Autodesk Fusion 360 part; units mm, degrees
(part 2 of 8)
  line L951 (106.594, 69.8334) -> (107.395, 69.8334)
  line L952 (107.395, 69.8334) -> (107.395, 64.0334)
  line L953 (107.395, 64.0334) -> (106.594, 64.0334)
  line L954 (106.594, 64.0334) -> (106.594, 60.9328)
  line L955 (106.594, 60.9328) -> (107.395, 60.9328)
  line L956 (107.395, 60.9328) -> (107.395, 59.9338)
  line L957 (107.395, 59.9338) -> (121.394, 59.9338)
  line L958 (121.394, 59.9338) -> (121.394, 60.9328)
  line L959 (121.394, 60.9328) -> (122.195, 60.9328)
  line L960 (122.195, 60.9328) -> (122.195, 64.0334)
  line L961 (122.195, 64.0334) -> (121.394, 64.0334)
  line L962 (121.394, 64.0334) -> (121.394, 69.8334)
  line L963 (121.394, 69.8334) -> (122.195, 69.8334)
  line L964 (122.195, 69.8334) -> (122.195, 72.9326)
  line L965 (122.195, 72.9326) -> (121.394, 72.9326)
  line L966 (121.394, 72.9326) -> (121.394, 73.9331)
  line L967 (121.394, 73.9331) -> (107.395, 73.9331)
  line L968 (126.445, 73.9331) -> (126.445, 72.9326)
  line L969 (126.445, 72.9326) -> (125.644, 72.9326)
  line L970 (125.644, 72.9326) -> (125.644, 69.8334)
  line L971 (125.644, 69.8334) -> (126.445, 69.8334)
  line L972 (126.445, 69.8334) -> (126.445, 64.0334)
  line L973 (126.445, 64.0334) -> (125.644, 64.0334)
  line L974 (125.644, 64.0334) -> (125.644, 60.9328)
  line L975 (125.644, 60.9328) -> (126.445, 60.9328)
  line L976 (126.445, 60.9328) -> (126.445, 59.9338)
  line L977 (126.445, 59.9338) -> (140.444, 59.9338)
  line L978 (140.444, 59.9338) -> (140.444, 60.9328)
  line L979 (140.444, 60.9328) -> (141.245, 60.9328)
  line L980 (141.245, 60.9328) -> (141.245, 64.0334)
  line L981 (141.245, 64.0334) -> (140.444, 64.0334)
  line L982 (140.444, 64.0334) -> (140.444, 69.8334)
  line L983 (140.444, 69.8334) -> (141.245, 69.8334)
  line L984 (141.245, 69.8334) -> (141.245, 72.9326)
  line L985 (141.245, 72.9326) -> (140.444, 72.9326)
  line L986 (140.444, 72.9326) -> (140.444, 73.9331)
  line L987 (140.444, 73.9331) -> (126.445, 73.9331)
  line L988 (145.495, 73.9331) -> (145.495, 72.9326)
  line L989 (145.495, 72.9326) -> (144.694, 72.9326)
  line L990 (144.694, 72.9326) -> (144.694, 69.8334)
  line L991 (144.694, 69.8334) -> (145.495, 69.8334)
  line L992 (145.495, 69.8334) -> (145.495, 64.0334)
  line L993 (145.495, 64.0334) -> (144.694, 64.0334)
  line L994 (144.694, 64.0334) -> (144.694, 60.9328)
  line L995 (144.694, 60.9328) -> (145.495, 60.9328)
  line L996 (145.495, 60.9328) -> (145.495, 59.9338)
  line L997 (145.495, 59.9338) -> (159.494, 59.9338)
  line L998 (159.494, 59.9338) -> (159.494, 60.9328)
  line L999 (159.494, 60.9328) -> (160.295, 60.9328)
  line L1000 (160.295, 60.9328) -> (160.295, 64.0334)
  line L1001 (160.295, 64.0334) -> (159.494, 64.0334)
  line L1002 (159.494, 64.0334) -> (159.494, 69.8334)
  line L1003 (159.494, 69.8334) -> (160.295, 69.8334)
  line L1004 (160.295, 69.8334) -> (160.295, 72.9326)
  line L1005 (160.295, 72.9326) -> (159.494, 72.9326)
  line L1006 (159.494, 72.9326) -> (159.494, 73.9331)
  line L1007 (159.494, 73.9331) -> (145.495, 73.9331)
  line L1008 (164.545, 73.9331) -> (164.545, 72.9326)
  line L1009 (164.545, 72.9326) -> (163.744, 72.9326)
  line L1010 (163.744, 72.9326) -> (163.744, 69.8334)
  line L1011 (163.744, 69.8334) -> (164.545, 69.8334)
  line L1012 (164.545, 69.8334) -> (164.545, 64.0334)
  line L1013 (164.545, 64.0334) -> (163.744, 64.0334)
  line L1014 (163.744, 64.0334) -> (163.744, 60.9328)
  line L1015 (163.744, 60.9328) -> (164.545, 60.9328)
  line L1016 (164.545, 60.9328) -> (164.545, 59.9338)
  line L1017 (164.545, 59.9338) -> (178.544, 59.9338)
  line L1018 (178.544, 59.9338) -> (178.544, 60.9328)
  line L1019 (178.544, 60.9328) -> (179.345, 60.9328)
  line L1020 (179.345, 60.9328) -> (179.345, 64.0334)
  line L1021 (179.345, 64.0334) -> (178.544, 64.0334)
  line L1022 (178.544, 64.0334) -> (178.544, 69.8334)
  line L1023 (178.544, 69.8334) -> (179.345, 69.8334)
  line L1024 (179.345, 69.8334) -> (179.345, 72.9326)
  line L1025 (179.345, 72.9326) -> (178.544, 72.9326)
  line L1026 (178.544, 72.9326) -> (178.544, 73.9331)
  line L1027 (178.544, 73.9331) -> (164.545, 73.9331)
  line L1028 (183.595, 73.9331) -> (183.595, 72.9326)
  line L1029 (183.595, 72.9326) -> (182.794, 72.9326)
  line L1030 (182.794, 72.9326) -> (182.794, 69.8334)
  line L1031 (182.794, 69.8334) -> (183.595, 69.8334)
  line L1032 (183.595, 69.8334) -> (183.595, 64.0334)
  line L1033 (183.595, 64.0334) -> (182.794, 64.0334)
  line L1034 (182.794, 64.0334) -> (182.794, 60.9328)
  line L1035 (182.794, 60.9328) -> (183.595, 60.9328)
  line L1036 (183.595, 60.9328) -> (183.595, 59.9338)
  line L1037 (183.595, 59.9338) -> (197.594, 59.9338)
  line L1038 (197.594, 59.9338) -> (197.594, 60.9328)
  line L1039 (197.594, 60.9328) -> (198.395, 60.9328)
  line L1040 (198.395, 60.9328) -> (198.395, 64.0334)
  line L1041 (198.395, 64.0334) -> (197.594, 64.0334)
  line L1042 (197.594, 64.0334) -> (197.594, 69.8334)
  line L1043 (197.594, 69.8334) -> (198.395, 69.8334)
  line L1044 (198.395, 69.8334) -> (198.395, 72.9326)
  line L1045 (198.395, 72.9326) -> (197.594, 72.9326)
  line L1046 (197.594, 72.9326) -> (197.594, 73.9331)
  line L1047 (197.594, 73.9331) -> (183.595, 73.9331)
  line L1048 (202.645, 73.9331) -> (202.645, 72.9326)
  line L1049 (202.645, 72.9326) -> (201.844, 72.9326)
  line L1050 (201.844, 72.9326) -> (201.844, 69.8334)
  line L1051 (201.844, 69.8334) -> (202.645, 69.8334)
  line L1052 (202.645, 69.8334) -> (202.645, 64.0334)
  line L1053 (202.645, 64.0334) -> (201.844, 64.0334)
  line L1054 (201.844, 64.0334) -> (201.844, 60.9328)
  line L1055 (201.844, 60.9328) -> (202.645, 60.9328)
  line L1056 (202.645, 60.9328) -> (202.645, 59.9338)
  line L1057 (202.645, 59.9338) -> (216.644, 59.9338)
  line L1058 (216.644, 59.9338) -> (216.644, 60.9328)
  line L1059 (216.644, 60.9328) -> (217.445, 60.9328)
  line L1060 (217.445, 60.9328) -> (217.445, 64.0334)
  line L1061 (217.445, 64.0334) -> (216.644, 64.0334)
  line L1062 (216.644, 64.0334) -> (216.644, 69.8334)
  line L1063 (216.644, 69.8334) -> (217.445, 69.8334)
  line L1064 (217.445, 69.8334) -> (217.445, 72.9326)
  line L1065 (217.445, 72.9326) -> (216.644, 72.9326)
  line L1066 (216.644, 72.9326) -> (216.644, 73.9331)
  line L1067 (216.644, 73.9331) -> (202.645, 73.9331)
  line L1068 (221.695, 73.9331) -> (221.695, 72.9326)
  line L1069 (221.695, 72.9326) -> (220.894, 72.9326)
  line L1070 (220.894, 72.9326) -> (220.894, 69.8334)
  line L1071 (220.894, 69.8334) -> (221.695, 69.8334)
  line L1072 (221.695, 69.8334) -> (221.695, 64.0334)
  line L1073 (221.695, 64.0334) -> (220.894, 64.0334)
  line L1074 (220.894, 64.0334) -> (220.894, 60.9328)
  line L1075 (220.894, 60.9328) -> (221.695, 60.9328)
  line L1076 (221.695, 60.9328) -> (221.695, 59.9338)
  line L1077 (221.695, 59.9338) -> (235.694, 59.9338)
  line L1078 (235.694, 59.9338) -> (235.694, 60.9328)
  line L1079 (235.694, 60.9328) -> (236.495, 60.9328)
  line L1080 (236.495, 60.9328) -> (236.495, 64.0334)
  line L1081 (236.495, 64.0334) -> (235.694, 64.0334)
  line L1082 (235.694, 64.0334) -> (235.694, 69.8334)
  line L1083 (235.694, 69.8334) -> (236.495, 69.8334)
  line L1084 (236.495, 69.8334) -> (236.495, 72.9326)
  line L1085 (236.495, 72.9326) -> (235.694, 72.9326)
  line L1086 (235.694, 72.9326) -> (235.694, 73.9331)
  line L1087 (235.694, 73.9331) -> (221.695, 73.9331)
  line L1088 (240.745, 73.9331) -> (240.745, 72.9326)
  line L1089 (240.745, 72.9326) -> (239.944, 72.9326)
  line L1090 (239.944, 72.9326) -> (239.944, 69.8334)
  line L1091 (239.944, 69.8334) -> (240.745, 69.8334)
  line L1092 (240.745, 69.8334) -> (240.745, 64.0334)
  line L1093 (240.745, 64.0334) -> (239.944, 64.0334)
  line L1094 (239.944, 64.0334) -> (239.944, 60.9328)
  line L1095 (239.944, 60.9328) -> (240.745, 60.9328)
  line L1096 (240.745, 60.9328) -> (240.745, 59.9338)
  line L1097 (240.745, 59.9338) -> (254.744, 59.9338)
  line L1098 (254.744, 59.9338) -> (254.744, 60.9328)
  line L1099 (254.744, 60.9328) -> (255.545, 60.9328)
  line L1100 (255.545, 60.9328) -> (255.545, 64.0334)
  line L1101 (255.545, 64.0334) -> (254.744, 64.0334)
  line L1102 (254.744, 64.0334) -> (254.744, 69.8334)
  line L1103 (254.744, 69.8334) -> (255.545, 69.8334)
  line L1104 (255.545, 69.8334) -> (255.545, 72.9326)
  line L1105 (255.545, 72.9326) -> (254.744, 72.9326)
  line L1106 (254.744, 72.9326) -> (254.744, 73.9331)
  line L1107 (254.744, 73.9331) -> (240.745, 73.9331)
  line L1108 (264.557, 73.9331) -> (264.557, 72.9326)
  line L1109 (264.557, 72.9326) -> (263.756, 72.9326)
  line L1110 (263.756, 72.9326) -> (263.756, 69.8334)
  line L1111 (263.756, 69.8334) -> (264.557, 69.8334)
  line L1112 (264.557, 69.8334) -> (264.557, 64.0334)
  line L1113 (264.557, 64.0334) -> (263.756, 64.0334)
  line L1114 (263.756, 64.0334) -> (263.756, 60.9328)
  line L1115 (263.756, 60.9328) -> (264.557, 60.9328)
  line L1116 (264.557, 60.9328) -> (264.557, 59.9338)
  line L1117 (264.557, 59.9338) -> (278.557, 59.9338)
  line L1118 (278.557, 59.9338) -> (278.557, 60.9328)
  line L1119 (278.557, 60.9328) -> (279.356, 60.9328)
  line L1120 (279.356, 60.9328) -> (279.356, 64.0334)
  line L1121 (279.356, 64.0334) -> (278.557, 64.0334)
  line L1122 (278.557, 64.0334) -> (278.557, 69.8334)
  line L1123 (278.557, 69.8334) -> (279.356, 69.8334)
  line L1124 (279.356, 69.8334) -> (279.356, 72.9326)
  line L1125 (279.356, 72.9326) -> (278.557, 72.9326)
  line L1126 (278.557, 72.9326) -> (278.557, 73.9331)
  line L1127 (278.557, 73.9331) -> (264.557, 73.9331)
  line L1128 (293.132, 73.9331) -> (293.132, 72.9326)
  line L1129 (293.132, 72.9326) -> (292.331, 72.9326)
  line L1130 (292.331, 72.9326) -> (292.331, 69.8334)
  line L1131 (292.331, 69.8334) -> (293.132, 69.8334)
  line L1132 (293.132, 69.8334) -> (293.132, 64.0334)
  line L1133 (293.132, 64.0334) -> (292.331, 64.0334)
  line L1134 (292.331, 64.0334) -> (292.331, 60.9328)
  line L1135 (292.331, 60.9328) -> (293.132, 60.9328)
  line L1136 (293.132, 60.9328) -> (293.132, 59.9338)
  line L1137 (293.132, 59.9338) -> (307.132, 59.9338)
  line L1138 (307.132, 59.9338) -> (307.132, 60.9328)
  line L1139 (307.132, 60.9328) -> (307.931, 60.9328)
  line L1140 (307.931, 60.9328) -> (307.931, 64.0334)
  line L1141 (307.931, 64.0334) -> (307.132, 64.0334)
  line L1142 (307.132, 64.0334) -> (307.132, 69.8334)
  line L1143 (307.132, 69.8334) -> (307.931, 69.8334)
  line L1144 (307.931, 69.8334) -> (307.931, 72.9326)
  line L1145 (307.931, 72.9326) -> (307.132, 72.9326)
  line L1146 (307.132, 72.9326) -> (307.132, 73.9331)
  line L1147 (307.132, 73.9331) -> (293.132, 73.9331)
  line L1148 (312.182, 73.9331) -> (312.182, 72.9326)
  line L1149 (312.182, 72.9326) -> (311.381, 72.9326)
  line L1150 (311.381, 72.9326) -> (311.381, 69.8334)
  line L1151 (311.381, 69.8334) -> (312.182, 69.8334)
  line L1152 (312.182, 69.8334) -> (312.182, 64.0334)
  line L1153 (312.182, 64.0334) -> (311.381, 64.0334)
  line L1154 (311.381, 64.0334) -> (311.381, 60.9328)
  line L1155 (311.381, 60.9328) -> (312.182, 60.9328)
  line L1156 (312.182, 60.9328) -> (312.182, 59.9338)
  line L1157 (312.182, 59.9338) -> (326.182, 59.9338)
  line L1158 (326.182, 59.9338) -> (326.182, 60.9328)
  line L1159 (326.182, 60.9328) -> (326.981, 60.9328)
  line L1160 (326.981, 60.9328) -> (326.981, 64.0334)
  line L1161 (326.981, 64.0334) -> (326.182, 64.0334)
  line L1162 (326.182, 64.0334) -> (326.182, 69.8334)
  line L1163 (326.182, 69.8334) -> (326.981, 69.8334)
  line L1164 (326.981, 69.8334) -> (326.981, 72.9326)
  line L1165 (326.981, 72.9326) -> (326.182, 72.9326)
  line L1166 (326.182, 72.9326) -> (326.182, 73.9331)
  line L1167 (326.182, 73.9331) -> (312.182, 73.9331)
  line L1168 (259.795, 92.9831) -> (259.795, 91.9826)
  line L1169 (259.795, 91.9826) -> (258.994, 91.9826)
  line L1170 (258.994, 91.9826) -> (258.994, 88.8834)
  line L1171 (258.994, 88.8834) -> (259.795, 88.8834)
  line L1172 (259.795, 88.8834) -> (259.795, 88.2826)
  line L1173 (259.795, 88.2826) -> (258.269, 88.2826)
  line L1174 (258.269, 88.2826) -> (258.269, 91.5127)
  line L1175 (258.269, 91.5127) -> (251.52, 91.5127)
  line L1176 (251.52, 91.5127) -> (251.52, 88.2826)
  line L1177 (251.52, 88.2826) -> (250.694, 88.2826)
  line L1178 (250.694, 88.2826) -> (250.694, 85.4837)
  line L1179 (250.694, 85.4837) -> (251.52, 85.4837)
  line L1180 (251.52, 85.4837) -> (251.52, 79.2138)
  line L1181 (251.52, 79.2138) -> (253.243, 79.2138)
  line L1182 (253.243, 79.2138) -> (253.243, 78.0136)
  line L1183 (253.243, 78.0136) -> (256.544, 78.0136)
  line L1184 (256.544, 78.0136) -> (256.544, 79.2138)
  line L1185 (256.544, 79.2138) -> (258.269, 79.2138)
  line L1186 (258.269, 79.2138) -> (258.269, 83.6828)
  line L1187 (258.269, 83.6828) -> (259.795, 83.6828)
  line L1188 (259.795, 83.6828) -> (259.795, 83.0834)
  line L1189 (259.795, 83.0834) -> (258.994, 83.0834)
  line L1190 (258.994, 83.0834) -> (258.994, 79.9828)
  line L1191 (258.994, 79.9828) -> (259.795, 79.9828)
  line L1192 (259.795, 79.9828) -> (259.795, 78.9838)
  line L1193 (259.795, 78.9838) -> (273.794, 78.9838)
  line L1194 (273.794, 78.9838) -> (273.794, 79.9828)
  line L1195 (273.794, 79.9828) -> (274.595, 79.9828)
  line L1196 (274.595, 79.9828) -> (274.595, 83.0834)
  line L1197 (274.595, 83.0834) -> (273.794, 83.0834)
  line L1198 (273.794, 83.0834) -> (273.794, 83.6828)
  line L1199 (273.794, 83.6828) -> (275.32, 83.6828)
  line L1200 (275.32, 83.6828) -> (275.32, 79.2138)
  line L1201 (275.32, 79.2138) -> (277.045, 79.2138)
  line L1202 (277.045, 79.2138) -> (277.045, 78.0136)
  line L1203 (277.045, 78.0136) -> (280.344, 78.0136)
  line L1204 (280.344, 78.0136) -> (280.344, 79.2138)
  line L1205 (280.344, 79.2138) -> (282.069, 79.2138)
  line L1206 (282.069, 79.2138) -> (282.069, 85.4837)
  line L1207 (282.069, 85.4837) -> (282.895, 85.4837)
  line L1208 (282.895, 85.4837) -> (282.895, 88.2826)
  line L1209 (282.895, 88.2826) -> (282.069, 88.2826)
  line L1210 (282.069, 88.2826) -> (282.069, 91.5127)
  line L1211 (282.069, 91.5127) -> (275.32, 91.5127)
  line L1212 (275.32, 91.5127) -> (275.32, 88.2826)
  line L1213 (275.32, 88.2826) -> (273.794, 88.2826)
  line L1214 (273.794, 88.2826) -> (273.794, 88.8834)
  line L1215 (273.794, 88.8834) -> (274.595, 88.8834)
  line L1216 (274.595, 88.8834) -> (274.595, 91.9826)
  line L1217 (274.595, 91.9826) -> (273.794, 91.9826)
  line L1218 (273.794, 91.9826) -> (273.794, 92.9831)
  line L1219 (273.794, 92.9831) -> (259.795, 92.9831)
  line L1220 (2.6197, 92.9831) -> (2.6197, 91.9826)
  line L1221 (2.6197, 91.9826) -> (1.819, 91.9826)
  line L1222 (1.819, 91.9826) -> (1.819, 88.8834)
  line L1223 (1.819, 88.8834) -> (2.6197, 88.8834)
  line L1224 (2.6197, 88.8834) -> (2.6197, 83.0834)
  line L1225 (2.6197, 83.0834) -> (1.819, 83.0834)
  line L1226 (1.819, 83.0834) -> (1.819, 79.9828)
  line L1227 (1.819, 79.9828) -> (2.6197, 79.9828)
  line L1228 (2.6197, 79.9828) -> (2.6197, 78.9838)
  line L1229 (2.6197, 78.9838) -> (16.6192, 78.9838)
  line L1230 (16.6192, 78.9838) -> (16.6192, 79.9828)
  line L1231 (16.6192, 79.9828) -> (17.4198, 79.9828)
  line L1232 (17.4198, 79.9828) -> (17.4198, 83.0834)
  line L1233 (17.4198, 83.0834) -> (16.6192, 83.0834)
  line L1234 (16.6192, 83.0834) -> (16.6192, 88.8834)
  line L1235 (16.6192, 88.8834) -> (17.4198, 88.8834)
  line L1236 (17.4198, 88.8834) -> (17.4198, 91.9826)
  line L1237 (17.4198, 91.9826) -> (16.6192, 91.9826)
  line L1238 (16.6192, 91.9826) -> (16.6192, 92.9831)
  line L1239 (16.6192, 92.9831) -> (2.6196, 92.9831)
  line L1240 (21.6697, 92.9831) -> (21.6697, 91.9826)
  line L1241 (21.6697, 91.9826) -> (20.869, 91.9826)
  line L1242 (20.869, 91.9826) -> (20.869, 88.8834)
  line L1243 (20.869, 88.8834) -> (21.6697, 88.8834)
  line L1244 (21.6697, 88.8834) -> (21.6697, 83.0834)
  line L1245 (21.6697, 83.0834) -> (20.869, 83.0834)
  line L1246 (20.869, 83.0834) -> (20.869, 79.9828)
  line L1247 (20.869, 79.9828) -> (21.6697, 79.9828)
  line L1248 (21.6697, 79.9828) -> (21.6697, 78.9838)
  line L1249 (21.6697, 78.9838) -> (35.669, 78.9838)
  line L1250 (35.669, 78.9838) -> (35.669, 79.9828)
  line L1251 (35.669, 79.9828) -> (36.4698, 79.9828)
  line L1252 (36.4698, 79.9828) -> (36.4698, 83.0834)
  line L1253 (36.4698, 83.0834) -> (35.669, 83.0834)
  line L1254 (35.669, 83.0834) -> (35.669, 88.8834)
  line L1255 (35.669, 88.8834) -> (36.4698, 88.8834)
  line L1256 (36.4698, 88.8834) -> (36.4698, 91.9826)
  line L1257 (36.4698, 91.9826) -> (35.669, 91.9826)
  line L1258 (35.669, 91.9826) -> (35.669, 92.9831)
  line L1259 (35.669, 92.9831) -> (21.6697, 92.9831)
  line L1260 (40.7197, 92.9831) -> (40.7197, 91.9826)
  line L1261 (40.7197, 91.9826) -> (39.9189, 91.9826)
  line L1262 (39.9189, 91.9826) -> (39.9189, 88.8834)
  line L1263 (39.9189, 88.8834) -> (40.7197, 88.8834)
  line L1264 (40.7197, 88.8834) -> (40.7197, 83.0834)
  line L1265 (40.7197, 83.0834) -> (39.9189, 83.0834)
  line L1266 (39.9189, 83.0834) -> (39.9189, 79.9828)
  line L1267 (39.9189, 79.9828) -> (40.7197, 79.9828)
  line L1268 (40.7197, 79.9828) -> (40.7197, 78.9838)
  line L1269 (40.7197, 78.9838) -> (54.719, 78.9838)
  line L1270 (54.719, 78.9838) -> (54.719, 79.9828)
  line L1271 (54.719, 79.9828) -> (55.5198, 79.9828)
  line L1272 (55.5198, 79.9828) -> (55.5198, 83.0834)
  line L1273 (55.5198, 83.0834) -> (54.719, 83.0834)
  line L1274 (54.719, 83.0834) -> (54.719, 88.8834)
  line L1275 (54.719, 88.8834) -> (55.5198, 88.8834)
  line L1276 (55.5198, 88.8834) -> (55.5198, 91.9826)
  line L1277 (55.5198, 91.9826) -> (54.719, 91.9826)
  line L1278 (54.719, 91.9826) -> (54.719, 92.9831)
  line L1279 (54.719, 92.9831) -> (40.7197, 92.9831)
  line L1280 (59.7697, 92.9831) -> (59.7697, 91.9826)
  line L1281 (59.7697, 91.9826) -> (58.9689, 91.9826)
  line L1282 (58.9689, 91.9826) -> (58.9689, 88.8834)
  line L1283 (58.9689, 88.8834) -> (59.7697, 88.8834)
  line L1284 (59.7697, 88.8834) -> (59.7697, 83.0834)
  line L1285 (59.7697, 83.0834) -> (58.9689, 83.0834)
  line L1286 (58.9689, 83.0834) -> (58.9689, 79.9828)
  line L1287 (58.9689, 79.9828) -> (59.7697, 79.9828)
  line L1288 (59.7697, 79.9828) -> (59.7697, 78.9838)
  line L1289 (59.7697, 78.9838) -> (73.769, 78.9838)
  line L1290 (73.769, 78.9838) -> (73.769, 79.9828)
  line L1291 (73.769, 79.9828) -> (74.5698, 79.9828)
  line L1292 (74.5698, 79.9828) -> (74.5698, 83.0834)
  line L1293 (74.5698, 83.0834) -> (73.769, 83.0834)
  line L1294 (73.769, 83.0834) -> (73.769, 88.8834)
  line L1295 (73.769, 88.8834) -> (74.5698, 88.8834)
  line L1296 (74.5698, 88.8834) -> (74.5698, 91.9826)
  line L1297 (74.5698, 91.9826) -> (73.769, 91.9826)
  line L1298 (73.769, 91.9826) -> (73.769, 92.9831)
  line L1299 (73.769, 92.9831) -> (59.7697, 92.9831)
  line L1300 (78.8197, 92.9831) -> (78.8197, 91.9826)
  line L1301 (78.8197, 91.9826) -> (78.0189, 91.9826)
  line L1302 (78.0189, 91.9826) -> (78.0189, 88.8834)
  line L1303 (78.0189, 88.8834) -> (78.8197, 88.8834)
  line L1304 (78.8197, 88.8834) -> (78.8197, 83.0834)
  line L1305 (78.8197, 83.0834) -> (78.0189, 83.0834)
  line L1306 (78.0189, 83.0834) -> (78.0189, 79.9828)
  line L1307 (78.0189, 79.9828) -> (78.8197, 79.9828)
  line L1308 (78.8197, 79.9828) -> (78.8197, 78.9838)
  line L1309 (78.8197, 78.9838) -> (92.819, 78.9838)
  line L1310 (92.819, 78.9838) -> (92.819, 79.9828)
  line L1311 (92.819, 79.9828) -> (93.6184, 79.9828)
  line L1312 (93.6184, 79.9828) -> (93.6184, 83.0834)
  line L1313 (93.6184, 83.0834) -> (92.819, 83.0834)
  line L1314 (92.819, 83.0834) -> (92.819, 88.8834)
  line L1315 (92.819, 88.8834) -> (93.6184, 88.8834)
  line L1316 (93.6184, 88.8834) -> (93.6184, 91.9826)
  line L1317 (93.6184, 91.9826) -> (92.819, 91.9826)
  line L1318 (92.819, 91.9826) -> (92.819, 92.9831)
  line L1319 (92.819, 92.9831) -> (78.8197, 92.9831)
  line L1320 (97.8683, 92.9831) -> (97.8683, 91.9826)
  line L1321 (97.8683, 91.9826) -> (97.0689, 91.9826)
  line L1322 (97.0689, 91.9826) -> (97.0689, 88.8834)
  line L1323 (97.0689, 88.8834) -> (97.8683, 88.8834)
  line L1324 (97.8683, 88.8834) -> (97.8683, 83.0834)
  line L1325 (97.8683, 83.0834) -> (97.0689, 83.0834)
  line L1326 (97.0689, 83.0834) -> (97.0689, 79.9828)
  line L1327 (97.0689, 79.9828) -> (97.8683, 79.9828)
  line L1328 (97.8683, 79.9828) -> (97.8683, 78.9838)
  line L1329 (97.8683, 78.9838) -> (111.869, 78.9838)
  line L1330 (111.869, 78.9838) -> (111.869, 79.9828)
  line L1331 (111.869, 79.9828) -> (112.668, 79.9828)
  line L1332 (112.668, 79.9828) -> (112.668, 83.0834)
  line L1333 (112.668, 83.0834) -> (111.869, 83.0834)
  line L1334 (111.869, 83.0834) -> (111.869, 88.8834)
  line L1335 (111.869, 88.8834) -> (112.668, 88.8834)
  line L1336 (112.668, 88.8834) -> (112.668, 91.9826)
  line L1337 (112.668, 91.9826) -> (111.869, 91.9826)
  line L1338 (111.869, 91.9826) -> (111.869, 92.9831)
  line L1339 (111.869, 92.9831) -> (97.8683, 92.9831)
  line L1340 (116.918, 92.9831) -> (116.918, 91.9826)
  line L1341 (116.918, 91.9826) -> (116.119, 91.9826)
  line L1342 (116.119, 91.9826) -> (116.119, 88.8834)
  line L1343 (116.119, 88.8834) -> (116.918, 88.8834)
  line L1344 (116.918, 88.8834) -> (116.918, 83.0834)
  line L1345 (116.918, 83.0834) -> (116.119, 83.0834)
  line L1346 (116.119, 83.0834) -> (116.119, 79.9828)
  line L1347 (116.119, 79.9828) -> (116.918, 79.9828)
  line L1348 (116.918, 79.9828) -> (116.918, 78.9838)
  line L1349 (116.918, 78.9838) -> (130.919, 78.9838)
  line L1350 (130.919, 78.9838) -> (130.919, 79.9828)
  line L1351 (130.919, 79.9828) -> (131.72, 79.9828)
  line L1352 (131.72, 79.9828) -> (131.72, 83.0834)
  line L1353 (131.72, 83.0834) -> (130.919, 83.0834)
  line L1354 (130.919, 83.0834) -> (130.919, 88.8834)
  line L1355 (130.919, 88.8834) -> (131.72, 88.8834)
  line L1356 (131.72, 88.8834) -> (131.72, 91.9826)
  line L1357 (131.72, 91.9826) -> (130.919, 91.9826)
  line L1358 (130.919, 91.9826) -> (130.919, 92.9831)
  line L1359 (130.919, 92.9831) -> (116.918, 92.9831)
  line L1360 (135.97, 92.9831) -> (135.97, 91.9826)
  line L1361 (135.97, 91.9826) -> (135.169, 91.9826)
  line L1362 (135.169, 91.9826) -> (135.169, 88.8834)
  line L1363 (135.169, 88.8834) -> (135.97, 88.8834)
  line L1364 (135.97, 88.8834) -> (135.97, 83.0834)
  line L1365 (135.97, 83.0834) -> (135.169, 83.0834)
  line L1366 (135.169, 83.0834) -> (135.169, 79.9828)
  line L1367 (135.169, 79.9828) -> (135.97, 79.9828)
  line L1368 (135.97, 79.9828) -> (135.97, 78.9838)
  line L1369 (135.97, 78.9838) -> (149.969, 78.9838)
  line L1370 (149.969, 78.9838) -> (149.969, 79.9828)
  line L1371 (149.969, 79.9828) -> (150.77, 79.9828)
  line L1372 (150.77, 79.9828) -> (150.77, 83.0834)
  line L1373 (150.77, 83.0834) -> (149.969, 83.0834)
  line L1374 (149.969, 83.0834) -> (149.969, 88.8834)
  line L1375 (149.969, 88.8834) -> (150.77, 88.8834)
  line L1376 (150.77, 88.8834) -> (150.77, 91.9826)
  line L1377 (150.77, 91.9826) -> (149.969, 91.9826)
  line L1378 (149.969, 91.9826) -> (149.969, 92.9831)
  line L1379 (149.969, 92.9831) -> (135.97, 92.9831)
  line L1380 (155.02, 92.9831) -> (155.02, 91.9826)
  line L1381 (155.02, 91.9826) -> (154.219, 91.9826)
  line L1382 (154.219, 91.9826) -> (154.219, 88.8834)
  line L1383 (154.219, 88.8834) -> (155.02, 88.8834)
  line L1384 (155.02, 88.8834) -> (155.02, 83.0834)
  line L1385 (155.02, 83.0834) -> (154.219, 83.0834)
  line L1386 (154.219, 83.0834) -> (154.219, 79.9828)
  line L1387 (154.219, 79.9828) -> (155.02, 79.9828)
  line L1388 (155.02, 79.9828) -> (155.02, 78.9838)
  line L1389 (155.02, 78.9838) -> (169.019, 78.9838)
  line L1390 (169.019, 78.9838) -> (169.019, 79.9828)
  line L1391 (169.019, 79.9828) -> (169.82, 79.9828)
  line L1392 (169.82, 79.9828) -> (169.82, 83.0834)
  line L1393 (169.82, 83.0834) -> (169.019, 83.0834)
  line L1394 (169.019, 83.0834) -> (169.019, 88.8834)
  line L1395 (169.019, 88.8834) -> (169.82, 88.8834)
  line L1396 (169.82, 88.8834) -> (169.82, 91.9826)
  line L1397 (169.82, 91.9826) -> (169.019, 91.9826)
  line L1398 (169.019, 91.9826) -> (169.019, 92.9831)
  line L1399 (169.019, 92.9831) -> (155.02, 92.9831)
  line L1400 (174.07, 92.9831) -> (174.07, 91.9826)
  line L1401 (174.07, 91.9826) -> (173.269, 91.9826)
  line L1402 (173.269, 91.9826) -> (173.269, 88.8834)
  line L1403 (173.269, 88.8834) -> (174.07, 88.8834)
  line L1404 (174.07, 88.8834) -> (174.07, 83.0834)
  line L1405 (174.07, 83.0834) -> (173.269, 83.0834)
  line L1406 (173.269, 83.0834) -> (173.269, 79.9828)
  line L1407 (173.269, 79.9828) -> (174.07, 79.9828)
  line L1408 (174.07, 79.9828) -> (174.07, 78.9838)
  line L1409 (174.07, 78.9838) -> (188.069, 78.9838)
  line L1410 (188.069, 78.9838) -> (188.069, 79.9828)
  line L1411 (188.069, 79.9828) -> (188.87, 79.9828)
  line L1412 (188.87, 79.9828) -> (188.87, 83.0834)
  line L1413 (188.87, 83.0834) -> (188.069, 83.0834)
  line L1414 (188.069, 83.0834) -> (188.069, 88.8834)
  line L1415 (188.069, 88.8834) -> (188.87, 88.8834)
  line L1416 (188.87, 88.8834) -> (188.87, 91.9826)
  line L1417 (188.87, 91.9826) -> (188.069, 91.9826)
  line L1418 (188.069, 91.9826) -> (188.069, 92.9831)
  line L1419 (188.069, 92.9831) -> (174.07, 92.9831)
  line L1420 (193.12, 92.9831) -> (193.12, 91.9826)
  line L1421 (193.12, 91.9826) -> (192.319, 91.9826)
  line L1422 (192.319, 91.9826) -> (192.319, 88.8834)
  line L1423 (192.319, 88.8834) -> (193.12, 88.8834)
  line L1424 (193.12, 88.8834) -> (193.12, 83.0834)
  line L1425 (193.12, 83.0834) -> (192.319, 83.0834)
  line L1426 (192.319, 83.0834) -> (192.319, 79.9828)
  line L1427 (192.319, 79.9828) -> (193.12, 79.9828)
  line L1428 (193.12, 79.9828) -> (193.12, 78.9838)
  line L1429 (193.12, 78.9838) -> (207.119, 78.9838)
  line L1430 (207.119, 78.9838) -> (207.119, 79.9828)
  line L1431 (207.119, 79.9828) -> (207.92, 79.9828)
  line L1432 (207.92, 79.9828) -> (207.92, 83.0834)
  line L1433 (207.92, 83.0834) -> (207.119, 83.0834)
  line L1434 (207.119, 83.0834) -> (207.119, 88.8834)
  line L1435 (207.119, 88.8834) -> (207.92, 88.8834)
  line L1436 (207.92, 88.8834) -> (207.92, 91.9826)
  line L1437 (207.92, 91.9826) -> (207.119, 91.9826)
  line L1438 (207.119, 91.9826) -> (207.119, 92.9831)
  line L1439 (207.119, 92.9831) -> (193.12, 92.9831)
  line L1440 (212.17, 92.9831) -> (212.17, 91.9826)
  line L1441 (212.17, 91.9826) -> (211.369, 91.9826)
  line L1442 (211.369, 91.9826) -> (211.369, 88.8834)
  line L1443 (211.369, 88.8834) -> (212.17, 88.8834)
  line L1444 (212.17, 88.8834) -> (212.17, 83.0834)
  line L1445 (212.17, 83.0834) -> (211.369, 83.0834)
  line L1446 (211.369, 83.0834) -> (211.369, 79.9828)
  line L1447 (211.369, 79.9828) -> (212.17, 79.9828)
  line L1448 (212.17, 79.9828) -> (212.17, 78.9838)
  line L1449 (212.17, 78.9838) -> (226.169, 78.9838)
  line L1450 (226.169, 78.9838) -> (226.169, 79.9828)
  line L1451 (226.169, 79.9828) -> (226.97, 79.9828)
  line L1452 (226.97, 79.9828) -> (226.97, 83.0834)
  line L1453 (226.97, 83.0834) -> (226.169, 83.0834)
  line L1454 (226.169, 83.0834) -> (226.169, 88.8834)
  line L1455 (226.169, 88.8834) -> (226.97, 88.8834)
  line L1456 (226.97, 88.8834) -> (226.97, 91.9826)
  line L1457 (226.97, 91.9826) -> (226.169, 91.9826)
  line L1458 (226.169, 91.9826) -> (226.169, 92.9831)
  line L1459 (226.169, 92.9831) -> (212.17, 92.9831)
  line L1460 (231.22, 92.9831) -> (231.22, 91.9826)
  line L1461 (231.22, 91.9826) -> (230.419, 91.9826)
  line L1462 (230.419, 91.9826) -> (230.419, 88.8834)
  line L1463 (230.419, 88.8834) -> (231.22, 88.8834)
  line L1464 (231.22, 88.8834) -> (231.22, 83.0834)
  line L1465 (231.22, 83.0834) -> (230.419, 83.0834)
  line L1466 (230.419, 83.0834) -> (230.419, 79.9828)
  line L1467 (230.419, 79.9828) -> (231.22, 79.9828)
  line L1468 (231.22, 79.9828) -> (231.22, 78.9838)
  line L1469 (231.22, 78.9838) -> (245.219, 78.9838)
  line L1470 (245.219, 78.9838) -> (245.219, 79.9828)
  line L1471 (245.219, 79.9828) -> (246.02, 79.9828)
  line L1472 (246.02, 79.9828) -> (246.02, 83.0834)
  line L1473 (246.02, 83.0834) -> (245.219, 83.0834)
  line L1474 (245.219, 83.0834) -> (245.219, 88.8834)
  line L1475 (245.219, 88.8834) -> (246.02, 88.8834)
  line L1476 (246.02, 88.8834) -> (246.02, 91.9826)
  line L1477 (246.02, 91.9826) -> (245.219, 91.9826)
  line L1478 (245.219, 91.9826) -> (245.219, 92.9831)
  line L1479 (245.219, 92.9831) -> (231.22, 92.9831)
  line L1480 (293.132, 92.9831) -> (293.132, 91.9826)
  line L1481 (293.132, 91.9826) -> (292.331, 91.9826)
  line L1482 (292.331, 91.9826) -> (292.331, 88.8834)
  line L1483 (292.331, 88.8834) -> (293.132, 88.8834)
  line L1484 (293.132, 88.8834) -> (293.132, 83.0834)
  line L1485 (293.132, 83.0834) -> (292.331, 83.0834)
  line L1486 (292.331, 83.0834) -> (292.331, 79.9828)
  line L1487 (292.331, 79.9828) -> (293.132, 79.9828)
  line L1488 (293.132, 79.9828) -> (293.132, 78.9838)
  line L1489 (293.132, 78.9838) -> (307.132, 78.9838)
  line L1490 (307.132, 78.9838) -> (307.132, 79.9828)
  line L1491 (307.132, 79.9828) -> (307.931, 79.9828)
  line L1492 (307.931, 79.9828) -> (307.931, 83.0834)
  line L1493 (307.931, 83.0834) -> (307.132, 83.0834)
  line L1494 (307.132, 83.0834) -> (307.132, 88.8834)
  line L1495 (307.132, 88.8834) -> (307.931, 88.8834)
  line L1496 (307.931, 88.8834) -> (307.931, 91.9826)
  line L1497 (307.931, 91.9826) -> (307.132, 91.9826)
  line L1498 (307.132, 91.9826) -> (307.132, 92.9831)
  line L1499 (307.132, 92.9831) -> (293.132, 92.9831)
  line L1500 (312.182, 92.9831) -> (312.182, 91.9826)
  line L1501 (312.182, 91.9826) -> (311.381, 91.9826)
  line L1502 (311.381, 91.9826) -> (311.381, 88.8834)
  line L1503 (311.381, 88.8834) -> (312.182, 88.8834)
  line L1504 (312.182, 88.8834) -> (312.182, 83.0834)
  line L1505 (312.182, 83.0834) -> (311.381, 83.0834)
  line L1506 (311.381, 83.0834) -> (311.381, 79.9828)
  line L1507 (311.381, 79.9828) -> (312.182, 79.9828)
  line L1508 (312.182, 79.9828) -> (312.182, 78.9838)
  line L1509 (312.182, 78.9838) -> (326.182, 78.9838)
  line L1510 (326.182, 78.9838) -> (326.182, 79.9828)
  line L1511 (326.182, 79.9828) -> (326.981, 79.9828)
  line L1512 (326.981, 79.9828) -> (326.981, 83.0834)
  line L1513 (326.981, 83.0834) -> (326.182, 83.0834)
  line L1514 (326.182, 83.0834) -> (326.182, 88.8834)
  line L1515 (326.182, 88.8834) -> (326.981, 88.8834)
  line L1516 (326.981, 88.8834) -> (326.981, 91.9826)
  line L1517 (326.981, 91.9826) -> (326.182, 91.9826)
  line L1518 (326.182, 91.9826) -> (326.182, 92.9831)
  line L1519 (326.182, 92.9831) -> (312.182, 92.9831)
  line L1520 (-13.3898, 113.6093) -> (346.941, 113.6093)
  line L1521 (346.941, 113.6093) -> (346.941, -14.3001)
  line L1522 (346.941, -14.3001) -> (-13.3898, -14.3001)
  line L1523 (-13.3898, -14.3001) -> (-13.3898, 113.6093)
  line L1524 (2.6197, 85.9834) -> (16.6192, 85.9834) construction
  line L1525 (9.6194, 92.9831) -> (9.6194, 78.9838) construction
  line L1526 (14.3819, 73.9331) -> (14.3819, 59.9338) construction
  line L1527 (7.3822, 66.9334) -> (21.3817, 66.9334) construction
  line L1528 (16.7625, 54.8831) -> (16.7625, 40.8838) construction
  line L1529 (9.762, 47.8834) -> (23.7629, 47.8834) construction
  line L1530 (21.5256, 35.833) -> (21.5256, 21.8336) construction
  line L1531 (33.4257, 34.3628) -> (33.425, 20.8635) construction
  line L1532 (9.6256, 34.3628) -> (9.6256, 20.8635) construction
  line L1533 (21.5256, 28.8333) -> (37.6259, 28.8333) construction
  line L1534 (21.5256, 28.8333) -> (5.4253, 28.8333) construction
  line L1535 (5.0009, 9.784) -> (19.0004, 9.784) construction
  line L1536 (12.0007, 16.7831) -> (12.0007, 2.7836) construction
  line L1537 (312.182, 85.9834) -> (326.182, 85.9834) construction
  line L1538 (319.182, 92.9831) -> (319.182, 78.9838) construction
  line L1539 (319.182, 73.9331) -> (319.182, 59.9338) construction
  line L1540 (312.182, 66.9334) -> (326.182, 66.9334) construction
  line L1541 (312.182, 9.784) -> (326.182, 9.784) construction
  line L1542 (319.182, 16.7831) -> (319.182, 2.7836) construction
  line L1543 (259.795, 91.9826) -> (259.795, 88.8834)
  line L1544 (259.795, 83.0834) -> (259.795, 79.9828)
  line L1545 (273.794, 83.0834) -> (273.794, 79.9828)
  line L1546 (273.794, 91.9826) -> (273.794, 88.8834)
  line L1547 (257.412, 53.8826) -> (257.412, 50.7834)
  line L1548 (271.413, 53.8826) -> (271.413, 50.7834)
  line L1549 (271.413, 44.9834) -> (271.413, 41.8828)
  line L1550 (257.412, 44.9834) -> (257.412, 41.8828)
  line L1551 (252.65, 34.8327) -> (252.65, 31.7348)
  line L1552 (252.65, 25.9333) -> (252.65, 22.8327)
  line L1553 (266.65, 34.8327) -> (266.65, 31.7348)
  line L1554 (266.65, 25.9333) -> (266.65, 22.8327)
  line L1555 (28.5254, 34.8327) -> (28.5254, 31.7348)
  line L1556 (14.5259, 34.8327) -> (14.5259, 31.7348)
  line L1557 (14.5259, 25.9333) -> (14.5259, 22.8327)
  line L1558 (28.5254, 25.9333) -> (28.5254, 22.8327)
  constraint horizontal L1520
  constraint vertical L1521
  constraint horizontal L1522
  constraint vertical L1523
  constraint midpoint L1224 L1524.start
  constraint midpoint L1234 L1524.end
  constraint midpoint L1239 L1525.start
  constraint midpoint L1229 L1525.end
  constraint perpendicular L1229 L1525
  constraint midpoint L867 L1526.start
  constraint midpoint L857 L1526.end
  constraint perpendicular L857 L1526
  constraint midpoint L852 L1527.start
  constraint midpoint L862 L1527.end
  constraint perpendicular L862 L1527
  constraint midpoint L627 L1528.start
  constraint midpoint L617 L1528.end
  constraint perpendicular L617 L1528
  constraint midpoint L612 L1529.start
  constraint midpoint L622 L1529.end
  constraint midpoint L283 L1530.start
  constraint midpoint L257 L1530.end
  constraint perpendicular L257 L1530
  constraint midpoint L275 L1531.start
  constraint midpoint L267 L1531.end
  constraint midpoint L239 L1532.start
  constraint midpoint L247 L1532.end
  constraint midpoint L1530 L1533.start
  constraint coincident L272 L1533.end
  constraint perpendicular L272 L1533
  constraint coincident L242 L1534.end
  constraint perpendicular L242 L1534
  constraint midpoint L56 L1535.start
  constraint midpoint L66 L1535.end
  constraint perpendicular L66 L1535
  constraint midpoint L71 L1536.start
  constraint midpoint L61 L1536.end
  constraint midpoint L1504 L1537.start
  constraint midpoint L1514 L1537.end
  constraint midpoint L1519 L1538.start
  constraint midpoint L1509 L1538.end
  constraint midpoint L1167 L1539.start
  constraint midpoint L1157 L1539.end
  constraint midpoint L1152 L1540.start
  constraint midpoint L1162 L1540.end
  constraint perpendicular L1162 L1540
  constraint midpoint L216 L1541.start
  constraint midpoint L226 L1541.end
  constraint midpoint L231 L1542.start
  constraint midpoint L221 L1542.end
  constraint perpendicular L221 L1542
  constraint perpendicular L1171 L1543
  constraint perpendicular L1191 L1544
  constraint perpendicular L1195 L1545
  constraint perpendicular L1215 L1546
  constraint perpendicular L559 L1547
  constraint perpendicular L603 L1548
  constraint perpendicular L583 L1549
  constraint perpendicular L579 L1550
  constraint perpendicular L287 L1551
  constraint perpendicular L307 L1552
  constraint perpendicular L333 L1553
  constraint perpendicular L311 L1554
  constraint perpendicular L279 L1555
  constraint perpendicular L235 L1556
  constraint perpendicular L255 L1557
  constraint perpendicular L259 L1558
sketch "Sketch3" plane through (0, 0, 0) normal (0, 0, 1) x (1, 0, 0)
  circle A0 centre (0.0007, 95.6021) radius 1.1
  line L0 (2.6197, 85.9834) -> (16.6192, 85.9834)
  circle A1 centre (0.0007, 0.259) radius 1.1
  line L1 (12.0007, 16.7831) -> (12.0007, 2.7836)
  circle A2 centre (328.707, 95.6021) radius 1.1
  circle A3 centre (328.707, 0.259) radius 1.1
  line L2 (319.182, 16.7831) -> (319.182, 2.7836)
  line L3 (312.182, 9.784) -> (326.182, 9.784)
  line L4 (0.0007, 95.6021) -> (328.707, 95.6021) construction
  line L5 (328.707, 95.6021) -> (328.707, 0.259) construction
  line L6 (328.707, 0.259) -> (0.0007, 0.259) construction
  line L7 (0.0007, 0.259) -> (0.0007, 95.6021) construction
  circle A4 centre (0.0007, 58.4334) radius 1.1
  circle A5 centre (328.707, 58.5271) radius 1.1
  circle A6 centre (287.1209, 77.5771) radius 1.1
  circle A7 centre (287.1209, 39.4771) radius 1.1
  line L8 (287.1209, 77.5771) -> (287.1209, 95.6021) construction
  line L9 (287.1209, 77.5771) -> (287.1209, 0.259) construction
  circle A8 centre (95.3444, 95.6021) radius 1.1
  circle A9 centre (171.5444, 95.6021) radius 1.1
  circle A10 centre (247.7444, 95.6021) radius 1.1
  circle A11 centre (69.1492, 0.259) radius 1.1
  circle A12 centre (192.9742, 0.259) radius 1.1
  circle A13 centre (259.6482, 0.259) radius 1.1
  line L10 (328.707, 58.5271) -> (0.0007, 58.4334) construction
  line L11 (287.1209, 39.4771) -> (0.0007, 39.4771) construction
  circle A14 centre (204.8826, 39.4771) radius 1.1
  circle A15 centre (128.6826, 39.4771) radius 1.1
  circle A16 centre (85.8193, 58.4579) radius 1.1
  circle A17 centre (162.0193, 58.4796) radius 1.1
  circle A18 centre (238.2193, 58.5013) radius 1.1
  point P0 (9.6194, 92.9831)
  dimension "d5" = 2.2
  dimension "d8" = 9.6187
  dimension "d9" = 9.6187
  dimension "d11" = 2.2
  dimension "d12" = 2.2
  dimension "d13" = 9.525
  dimension "d14" = 9.525
  dimension "d15" = 2.2
  dimension "d16" = 2.2
  dimension "d17" = 37.1687
  dimension "d18" = 37.075
  dimension "d19" = 2.2
  dimension "d20" = 41.5861
  dimension "d21" = 18.025
  dimension "d22" = 38.1
  dimension "d23" = 2.2
  dimension "d24" = 2.2
  dimension "d25" = 95.3437
  dimension "d26" = 76.2
  dimension "d27" = 76.2
  dimension "d28" = 69.1484
  dimension "d29" = 123.825
  dimension "d30" = 66.674
  dimension "d31" = 2.2
  dimension "d32" = 2.2
  dimension "d33" = 2.2
  dimension "d34" = 2.2
  dimension "d35" = 2.2
  dimension "d36" = 2.2
  dimension "d37" = 85.8186
  dimension "d38" = 76.2
  dimension "d39" = 76.2
  dimension "d40" = 128.6818
  dimension "d41" = 76.2
  dimension "d42" = 2.2
  dimension "d43" = 2.2
  dimension "d44" = 2.2
  dimension "d45" = 2.2
  dimension "d46" = 2.2
  constraint horizontal L4
  constraint vertical L5
  constraint horizontal L6
  constraint vertical L7
  constraint coincident A3.centre L5.end
  constraint coincident A0.centre L4.start
  constraint coincident A1.centre L6.end
  constraint coincident A2.centre L4.end
  constraint coincident L7 A4.centre
  constraint coincident L5 A5.centre
  constraint coincident A6.centre L8.start
  constraint coincident L4 L8.end
  constraint perpendicular L4 L8
  constraint coincident L6 L9.end
  constraint perpendicular L6 L9
  constraint coincident A7.centre L9
  constraint coincident L4 A10.centre
  constraint coincident L4 A9.centre
  constraint coincident L4 A8.centre
  constraint coincident L6 A11.centre
  constraint coincident L6 A12.centre
  constraint coincident L6 A13.centre
  constraint coincident A5.centre L10.start
  constraint coincident A4.centre L10.end
  constraint coincident A7.centre L11.start
  constraint coincident L7 L11.end
  constraint perpendicular L7 L11
  constraint coincident L10 A16.centre
  constraint coincident L10 A17.centre
  constraint coincident L11 A15.centre
  constraint coincident L11 A14.centre
  constraint coincident L10 A18.centre
  measures "d5" diameter of A0
  measures "d8" distance of A0.centre L0
  measures "d9" horizontal distance of A0.centre P0
  measures "d11" diameter of A1
  measures "d12" diameter of A2
  measures "d13" distance of A3.centre L2
  measures "d14" distance of A3.centre L3
  measures "d15" diameter of A3
  measures "d16" diameter of A4
  measures "d17" distance of A0.centre A4.centre
  measures "d18" distance of A2.centre A5.centre
  measures "d19" diameter of A5
  measures "d20" horizontal distance of A2.centre A6.centre
  measures "d21" vertical distance of A2.centre A6.centre
  measures "d22" distance of A6.centre A7.centre
  measures "d23" diameter of A7
  measures "d24" diameter of A6
  measures "d25" distance of A0.centre A8.centre
  measures "d26" distance of A8.centre A9.centre
  measures "d27" distance of A9.centre A10.centre
  measures "d28" distance of A1.centre A11.centre
  measures "d29" distance of A11.centre A12.centre
  measures "d30" distance of A12.centre A13.centre
  measures "d31" diameter of A13
  measures "d32" diameter of A12
  measures "d33" diameter of A11
  measures "d34" diameter of A8
  measures "d35" diameter of A9
  measures "d36" diameter of A10
  measures "d37" horizontal distance of A4.centre A16.centre
  measures "d38" horizontal distance of A16.centre A17.centre
  measures "d39" horizontal distance of A17.centre A18.centre
  measures "d40" distance of L11.end A15.centre
  measures "d41" distance of A14.centre A15.centre
  measures "d42" diameter of A16
  measures "d43" diameter of A17
  measures "d44" diameter of A18
  measures "d45" diameter of A14
  measures "d46" diameter of A15
sketch "Sketch4" plane through (0, 0, 0) normal (0, 0, 1) x (1, 0, 0)
  line L0 (0.0007, 98.0521) -> (328.707, 98.0521)
  line L1 (331.157, 95.6021) -> (331.157, 0.259)
  line L2 (328.707, -2.191) -> (0.0007, -2.191)
  line L3 (-2.4493, 0.259) -> (-2.4493, 95.6021)
  arc A0 (0.0007, 98.0521) -> (-2.4493, 95.6021) centre (0.0007, 95.6021) ccw
  arc A1 (-2.4493, 0.259) -> (0.0007, -2.191) centre (0.0007, 0.259) ccw
  arc A2 (328.707, -2.191) -> (331.157, 0.259) centre (328.707, 0.259) ccw
  arc A3 (331.157, 95.6021) -> (328.707, 98.0521) centre (328.707, 95.6021) ccw
  point P0 (0.0007, 95.6021)
  point P1 (0.0007, 0.259)
  point P2 (328.707, 0.259)
  dimension "d47" = 2.45
  dimension "d48" = 2.45
  dimension "d49" = 2.45
  dimension "d50" = 2.45
  dimension "d51" = 2.45
  constraint horizontal L0
  constraint vertical L1
  constraint horizontal L2
  constraint vertical L3
  constraint tangent L0 A0
  constraint tangent L3 A0
  constraint tangent L3 A1
  constraint tangent L2 A1
  constraint equal A0 A1
  constraint tangent L2 A2
  constraint tangent L1 A2
  constraint equal A0 A2
  constraint tangent L1 A3
  constraint tangent L0 A3
  constraint equal A0 A3
  measures "d47" distance of L0 P0
  measures "d48" distance of L3 P0
  measures "d49" distance of L2 P1
  measures "d50" distance of L1 P2
  measures "d51" radius of A0
extrude "Extrude1" add sketch "Sketch4" against normal blind 3